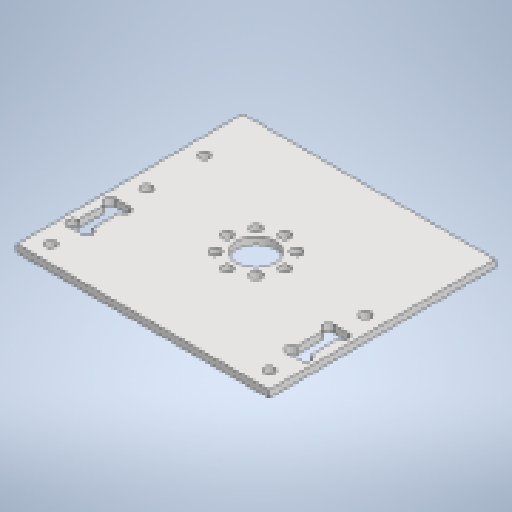
# Autodesk Inventor part: kosi_v3_1.5
Saved by Autodesk Inventor 2025.1 (Build 291241000, 241)
## iProperties
Created: 2024-09-01
Part Number: kosi_v3_1.5
Material: アルミニウム 2014-T4
Document SubType Name: Modeling
Designer: right
Density: 2.8 g/cm^3
Appearance: サテン
Mass: 9.61455 g
Surface Area: 51.3725 cm^2
Volume: 3.43377 cm^3
Author: right
Autodesk Inventor part; units mm, degrees
ref_plane "YZ Plane" through (0, 0, 0) normal (1, 0, 0) x (0, 1, 0)
ref_plane "XZ Plane" through (0, 0, 0) normal (0, 1, 0) x (-1, 0, 0)
ref_plane "XY Plane" through (0, 0, 0) normal (0, 0, 1) x (1, 0, 0)
sketch "スケッチ1" plane through (0, 0, 0) normal (0, 1, 0) x (-1, 0, 0)
  circle A0 centre (0, 0) radius 4
  circle A1 centre (0, 0) radius 8
  circle A2 centre (0, 0) radius 6 construction
  circle A3 centre (0, -6) radius 1.1
  circle A4 centre (4.2426, -4.2426) radius 1.1
  circle A5 centre (6, 0) radius 1.1
  circle A6 centre (4.2426, 4.2426) radius 1.1
  circle A7 centre (0, 6) radius 1.1
  circle A8 centre (-4.2426, 4.2426) radius 1.1
  circle A9 centre (-6, 0) radius 1.1
  circle A10 centre (-4.2426, -4.2426) radius 1.1
  line L0 (26.25, -23.5) -> (-26.25, -23.5)
  line L1 (-26.25, -23.5) -> (-26.25, 23.5)
  line L2 (-26.25, 23.5) -> (26.25, 23.5)
  line L3 (26.25, 23.5) -> (26.25, -23.5)
  line L4 (26.25, -23.5) -> (-26.25, 23.5) construction
  line L5 (-26.25, -23.5) -> (26.25, 23.5) construction
  line L6 (24.25, 5) -> (21.25, 5)
  line L7 (21.25, 5) -> (21.25, 15)
  line L8 (21.25, 15) -> (24.25, 15)
  line L9 (24.25, 15) -> (24.25, 5)
  circle A11 centre (24.25, 6.1) radius 1.1
  circle A12 centre (21.25, 6.1) radius 1.1
  line L10 (0, 0) -> (0, -23.5) construction
  circle A13 centre (24.25, 13.9) radius 1.1
  circle A14 centre (21.25, 13.9) radius 1.1
  line L11 (-24.25, 5) -> (-21.25, 5)
  line L12 (-21.25, 5) -> (-21.25, 15)
  line L13 (-21.25, 15) -> (-24.25, 15)
  line L14 (-24.25, 15) -> (-24.25, 5)
  circle A15 centre (-24.25, 6.1) radius 1.1
  circle A16 centre (-21.25, 6.1) radius 1.1
  circle A17 centre (-24.25, 13.9) radius 1.1
  circle A18 centre (-21.25, 13.9) radius 1.1
  circle A19 centre (22.75, 0) radius 1.1
  circle A20 centre (22.75, 20) radius 1.1
  circle A21 centre (-22.75, 0) radius 1.1
  circle A22 centre (-22.75, 20) radius 1.1
  circle A23 centre (22.75, 20) radius 3.5 construction
  point P0 (21.25, 10)
  point P1 (-21.25, 10)
  point P2 (22.75, 5)
  point P3 (-21.25, 12.8)
  point P4 (-21.25, 7.2)
  point P5 (-24.25, 7.2)
  point P6 (-24.25, 12.8)
  point P7 (-24.25, 15)
  point P8 (21.25, 12.8)
  point P9 (21.25, 15)
  point P10 (24.25, 15)
  point P11 (24.25, 12.8)
  point P12 (24.25, 7.2)
  point P13 (21.25, 7.2)
  point P14 (22.75, 15)
  dimension "d2" = 12
  dimension "d10" = 2.2
  dimension "d0" = 8
  dimension "d1" = 16
  dimension "d3" = 2.2
  dimension "d6" = 360
  dimension "d8" = 3
  dimension "d9" = 10
  dimension "d11" = 42.5
  dimension "d12" = 2.2
  dimension "d13" = 5
  dimension "d17" = 5
  dimension "d18" = 7
  constraints: 30 end point, 19 centre point, 11 symmetric about line, 7 midpoint, 6 point on line, 4 coincident, 4 parallel, 4 tangent, 4 vertical alignment, 2 equal radius, 2 horizontal, 2 perpendicular, 2 vertical, 1 horizontal alignment, 36 other
  measures "d0" diameter of A0
  measures "d1" diameter of A1
  measures "d3" diameter of A3
  measures "d8" distance of L6.start L6.end
  measures "d9" distance of L6.end L7.end
  measures "d11" distance between parallel lines of L12 L7
  measures "d12" diameter of A19
  measures "d13" distance from line of L6 A19.centre
  measures "d17" distance of point (22.75, 15) A20.centre
  measures "d18" diameter of A23
extrude "押し出し1" add sketch "スケッチ1" along normal blind 1.5 contours A1 | L0 L1 L2 L3
sketch "スケッチ2" plane through (0, 0, 0) normal (0, -1, 0) x (1, 0, 0)
  circle A0 centre (-22.75, -12) radius 1.1
  circle A1 centre (-22.75, 0) radius 1.1 projected
  point P0 (0, 0)
  dimension "d19" = 2.2
  dimension "d20" = 12
  constraints: 1 centre point, 1 vertical alignment
  measures "d19" diameter of A0
  measures "d20" distance of A0.centre A1.centre
extrude "押し出し2" cut sketch "スケッチ2" against normal through all contours A0
fillet "フィレット1" radius 2 4 edges at (-26.25, 0.75, -23.5) (26.25, 0.75, -23.5) (26.25, 0.75, 23.5) (-26.25, 0.75, 23.5)
equation "\"d17\" = d13"
